Autodesk Fusion 360 part; units mm, degrees
(part 2 of 2)
sketch "Right-Holders" plane through (0, 0, 0) normal (0, 0, 1) x (1, 0, 0)
  circle A0 centre (41.975, 135.062) radius 1.2
  circle A1 centre (70.837, 135.062) radius 1.2
  circle A2 centre (90.837, 135.062) radius 1.2
  circle A3 centre (41.975, 8) radius 1.2
  circle A4 centre (140.988, 8) radius 1.2
  circle A5 centre (161.325, 135.062) radius 1.2
  circle A6 centre (181.325, 135.062) radius 1.2
  circle A7 centre (241.4142, 134.4767) radius 1.2
  circle A8 centre (241.4142, 8.5858) radius 1.2
  line L0 (70.837, 131.062) -> (71.837, 131.062)
  line L1 (72.837, 132.062) -> (72.837, 133.062)
  line L2 (90.837, 131.062) -> (89.837, 131.062)
  line L3 (88.837, 132.062) -> (88.837, 133.062)
  line L4 (87.837, 134.062) -> (73.837, 134.062)
  line L5 (70.837, 131.062) -> (70.837, 130.062)
  line L6 (70.837, 130.062) -> (90.837, 130.062)
  line L7 (90.837, 130.062) -> (90.837, 131.062)
  arc A9 (73.837, 134.062) -> (72.837, 133.062) centre (73.837, 133.062) ccw
  arc A10 (71.837, 131.062) -> (72.837, 132.062) centre (71.837, 132.062) ccw
  arc A11 (88.837, 133.062) -> (87.837, 134.062) centre (87.837, 133.062) ccw
  arc A12 (88.837, 132.062) -> (89.837, 131.062) centre (89.837, 132.062) ccw
  line L8 (161.325, 131.062) -> (162.325, 131.062)
  line L9 (163.325, 132.062) -> (163.325, 133.062)
  line L10 (181.325, 131.062) -> (180.325, 131.062)
  line L11 (179.325, 132.062) -> (179.325, 133.062)
  line L12 (178.325, 134.062) -> (164.325, 134.062)
  line L13 (161.325, 131.062) -> (161.325, 130.062)
  line L14 (161.325, 130.062) -> (181.325, 130.062)
  line L15 (181.325, 130.062) -> (181.325, 131.062)
  arc A13 (164.325, 134.062) -> (163.325, 133.062) centre (164.325, 133.062) ccw
  arc A14 (162.325, 131.062) -> (163.325, 132.062) centre (162.325, 132.062) ccw
  arc A15 (179.325, 133.062) -> (178.325, 134.062) centre (178.325, 133.062) ccw
  arc A16 (179.325, 132.062) -> (180.325, 131.062) centre (180.325, 132.062) ccw
  point P0 (41.975, 135.062)
  point P1 (70.837, 135.062)
  point P2 (90.837, 135.062)
  point P3 (41.975, 8)
  point P4 (140.988, 8)
  point P5 (161.325, 135.062)
  point P6 (181.325, 135.062)
  point P7 (72.837, 131.062)
  point P8 (72.837, 134.062)
  point P9 (88.837, 131.062)
  point P10 (88.837, 134.062)
  point P11 (163.325, 131.062)
  point P12 (163.325, 134.062)
  point P13 (179.325, 131.062)
  point P14 (179.325, 134.062)
  dimension "d288" = 2.4
  dimension "d289" = 2.4
  dimension "d290" = 2.4
  dimension "d291" = 2.4
  dimension "d292" = 2.4
  dimension "d293" = 2.4
  dimension "d294" = 2.4
  dimension "d295" = 4
  dimension "d296" = 2
  dimension "d297" = 3
  dimension "d298" = 4
  dimension "d299" = 2
  dimension "d300" = 3
  dimension "d301" = 1
  dimension "d302" = 20
  dimension "d303" = 1
  dimension "d304" = 1
  dimension "d305" = 1
  dimension "d306" = 1
  dimension "d307" = 4
  dimension "d308" = 2
  dimension "d309" = 3
  dimension "d310" = 4
  dimension "d311" = 2
  dimension "d312" = 3
  dimension "d313" = 1
  dimension "d314" = 20
  dimension "d315" = 1
  dimension "d316" = 1
  dimension "d317" = 1
  dimension "d318" = 1
  dimension "d341" = 2.4
  dimension "d342" = 2.4
  constraint coincident P0 A0.centre
  constraint coincident P1 A1.centre
  constraint coincident P2 A2.centre
  constraint coincident P3 A3.centre
  constraint coincident P4 A4.centre
  constraint coincident P5 A5.centre
  constraint coincident P6 A6.centre
  constraint perpendicular L0 L1
  constraint perpendicular L2 L3
  constraint perpendicular L1 L4
  constraint perpendicular L0 L5
  constraint perpendicular L5 L6
  constraint perpendicular L2 L7
  constraint coincident P8 L1
  constraint coincident P8 L4
  constraint tangent L1 A9
  constraint tangent L4 A9
  constraint coincident P7 L0
  constraint coincident P7 L1
  constraint tangent L0 A10
  constraint tangent L1 A10
  constraint coincident P10 L3
  constraint coincident P10 L4
  constraint tangent L3 A11
  constraint tangent L4 A11
  constraint coincident P9 L2
  constraint coincident P9 L3
  constraint tangent L2 A12
  constraint tangent L3 A12
  constraint perpendicular L8 L9
  constraint perpendicular L10 L11
  constraint perpendicular L8 L13
  constraint perpendicular L13 L14
  constraint perpendicular L10 L15
  constraint coincident P12 L9
  constraint coincident P12 L12
  constraint tangent L9 A13
  constraint tangent L12 A13
  constraint coincident P11 L8
  constraint coincident P11 L9
  constraint tangent L8 A14
  constraint tangent L9 A14
  constraint coincident P14 L11
  constraint coincident P14 L12
  constraint tangent L11 A15
  constraint tangent L12 A15
  constraint coincident P13 L10
  constraint coincident P13 L11
  constraint tangent L10 A16
  constraint tangent L11 A16
  measures "d288" diameter of A0
  measures "d289" diameter of A1
  measures "d290" diameter of A2
  measures "d291" diameter of A3
  measures "d292" diameter of A4
  measures "d293" diameter of A5
  measures "d294" diameter of A6
  measures "d295" distance of P1 L0.start
  measures "d296" distance of L0.start P7
  measures "d297" distance of P7 P8
  measures "d298" distance of P2 L2.start
  measures "d299" distance of L2.start P9
  measures "d300" distance of P9 P10
  measures "d301" distance of L0.start L5.end
  measures "d302" distance of L5.end L6.end
  measures "d303" radius of A9
  measures "d304" radius of A10
  measures "d305" radius of A11
  measures "d306" radius of A12
  measures "d307" distance of P5 L8.start
  measures "d308" distance of L8.start P11
  measures "d309" distance of P11 P12
  measures "d310" distance of P6 L10.start
  measures "d311" distance of L10.start P13
  measures "d312" distance of P13 P14
  measures "d313" distance of L8.start L13.end
  measures "d314" distance of L13.end L14.end
  measures "d315" radius of A13
  measures "d316" radius of A14
  measures "d317" radius of A15
  measures "d318" radius of A16
  measures "d341" diameter of A7
  measures "d342" diameter of A8
extrude "Extrude-Top (1)" add sketch "Right-Main" along normal blind 1.8 from surface at 10.9 separate body contours L0 L1 L2 L12 L13 L14 L15 L23 A0 A1 makes body 2
extrude "Extrude-Side (1)" add sketch "Right-Main" along normal blind 11 from surface at 1.7 contours L3 L4 L5 L6 L7 L8 L9 L10 L11 L15 L16 L17 L18 L19 L20 L21 L22 L23 A2 A3 A4 A5 A6 A7 A8 A9 A10 A11 A12 A13 A14 A15 A16 A17 A18 A19 bodies 2
extrude "Extrude-Side2 (1)" add sketch "Right-Bottom" along normal blind 12.7 contours L0 L1 L2 L3 L4 L5 L6 L7 A0 A1 A2 A3 A4 A5 bodies 2
extrude "Extrude-Holder (1)" add sketch "Right-Bottom" along normal blind 11 from surface at 1.7 contours L3 L8 L9 L10 A6 | L3 L11 L12 A7 A8 | L5 L17 L18 L19 A11 | L3 L4 A5 L13 L14 A9 | L5 L20 L21 L22 A12 A13 | L5 L23 L24 L25 A14 A15 | L4 L5 A3 L15 L16 A10 bodies 2
extrude "Cut-Screw-Holes (1)" cut sketch "Right-Holders" along normal blind 15 bodies 2
extrude "Cut-USB-through (1)" cut sketch "Right-USB" along normal blind 20 from surface at 130 contours L0 A0 L1 A1 | L6 A4 L7 A5 bodies 2
extrude "Cut-USB-Out (1)" cut sketch "Right-USB" along normal blind 15 from surface at 137.043 contours L0 A0 A1 L3 A2 A3 L21 L22 L24 L25 A8 A9 | A0 L1 A1 A2 L4 A3 L21 L22 L24 L25 A8 A9 | L6 A4 A5 L9 A6 A7 L13 L14 L16 L18 A10 A11 | A4 L7 A5 A6 L10 A7 L13 L14 L16 L18 A10 A11 bodies 2
extrude "Cut-USB-In (1)" cut sketch "Right-USB" along normal blind 3.5 from surface at 132.063 contours L0 A0 A1 L3 A2 A3 L21 L22 L24 L25 A8 A9 | L3 A2 A3 L22 L23 L24 | L6 A4 A5 L9 A6 A7 L13 L14 L16 L18 A10 A11 | L9 A6 A7 L14 L15 L16 bodies 2
named bodies: "Left", "Right"
